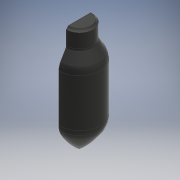
# Autodesk Inventor part: noze-cone
Saved by Autodesk Inventor 2017 (Build 210142000, 142)
## iProperties
Created: 2020-06-18
Part Number: noze-cone
Material: ABS Plastic
Document SubType Name: Modeling
Designer: HAYNIE R&D
Density: 1.06 g/cm^3
Appearance: Smooth - White
Author: HAYNIE R&D
Autodesk Inventor part; units mm, degrees
ref_plane "YZ Plane" through (0, 0, 0) normal (1, 0, 0) x (0, 1, 0)
ref_plane "XZ Plane" through (0, 0, 0) normal (0, 1, 0) x (-1, 0, 0)
ref_plane "XY Plane" through (0, 0, 0) normal (0, 0, 1) x (1, 0, 0)
sketch "Sketch1" plane through (0, 0, 0) normal (1, 0, 0) x (0, 1, 0)
  line L0 (0, 0) -> (0, -160)
  line L1 (17.75, -33.271) -> (27.75, -50.5915)
  line L2 (27.75, -50.5915) -> (27.75, -125.5915)
  arc A0 (0, -160) -> (27.75, -125.5915) centre (-66.0976, -78.299) ccw
  line L3 (0, -160) -> (0, -159)
  line L4 (16.75, -33.271) -> (26.75, -50.5915)
  line L5 (16.75, -33.271) -> (36.75, -33.271) construction
  line L6 (26.75, -50.5915) -> (26.75, -125.5915)
  arc A1 (0, -159) -> (26.75, -125.5915) centre (-67.3011, -77.6989) ccw
  line L7 (17.75, -33.271) -> (17.75, -13.271)
  line L8 (16.75, -13.271) -> (32.074, -13.271) construction
  line L9 (17.75, -13.271) -> (33.074, -13.271) construction
  line L10 (17.75, -13.271) -> (33.074, -13.271) construction
  line L11 (16.75, -13.271) -> (31.4966, -13.271) construction
  line L12 (16.75, -33.271) -> (16.75, -14.271)
  line L13 (16.75, -14.271) -> (0, -14.271)
  line L14 (17.75, -13.271) -> (0, -13.271)
  point P0 (0, -1)
  dimension "d0" = 160
  dimension "d7" = 75
  dimension "d15" = 1
  dimension "d31" = 19
  constraints: 30 end point, 5 horizontal, 5 point on line, 5 vertical, 4 point on circle, 2 centre point, 1 equal length, 1 perpendicular
  measures "d0" distance of L0.start L0.end
  measures "d7" distance of L1.end L2.end
  measures "d15" distance of L0.end L3.end
  measures "d31" distance of L4.start L12.end
revolve "Revolution2" add sketch "Sketch1" angle 360 about axis through (0, 0, 0) along (0, 0, -1) contours L14 L7 L1 L2 A0 L0 A1 L6 L4 L12 L13
fillet "Fillet5" radius 5 1 edges at (0, -17.75, -33.271)
sketch "Sketch4" plane through (0, 0, -13.271) normal (0, 0, 1) x (1, 0, 0)
  circle A0 centre (0, 0) radius 15
  dimension "d36" = 30
  constraints: 1 centre point, 1 coincident
  measures "d36" diameter of A0
extrude "Extrusion2" add sketch "Sketch4" along normal blind 3.27
split "Split3" plane through (0, 0, 0) removes the side toward (-1, 0, 0)
fillet "Fillet8" radius 20 1 edges at (27.75, 0, -50.5915)
fillet "Fillet9" radius 25 1 edges at (27.75, 0, -125.5915)
fillet "Fillet10" radius 10 1 edges at (15, 0, -13.271)
body "Solid2"
